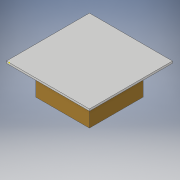
# Autodesk Inventor part: PartStoreipt
Saved by Autodesk Inventor 2018 (Build 220112000, 112)
## iProperties
Created: 2018-06-08
Part Number: PartStoreipt
Material: Generic
Document SubType Name: Modeling
Designer: 3400746
Density: 1 g/cm^3
Appearance: Default
Author: 3400746
Autodesk Inventor part; units mm, degrees
ref_plane "YZ Plane" through (0, 0, 0) normal (1, 0, 0) x (0, 1, 0)
ref_plane "XZ Plane" through (0, 0, 0) normal (0, 1, 0) x (-1, 0, 0)
ref_plane "XY Plane" through (0, 0, 0) normal (0, 0, 1) x (1, 0, 0)
sketch "Sketch1" plane through (0, 0, 0) normal (0, 1, 0) x (-1, 0, 0)
  line L0 (0, 0) -> (2159, 0)
  line L1 (2159, 0) -> (2159, -2159)
  line L2 (2159, -2159) -> (0, -2159)
  line L3 (0, -2159) -> (0, 0)
  dimension "d0" = 2159
  dimension "d1" = 2159
  dimension "d2" = 2159
  constraints: 8 end point, 2 perpendicular, 1 horizontal
  measures "d0" distance of L0.start L0.end
  measures "d1" distance of L0.end L1.end
  measures "d2" distance of L1.end L2.end
extrude "Extrusion1" add sketch "Sketch1" against normal blind 50.8
sketch "Sketch2" plane through (0, -50.8, 0) normal (0, -1, 0) x (1, 0, 0)
  line L0 (0, 0) -> (-2159, 0) projected
  line L1 (0, 0) -> (0, -381)
  line L2 (0, -2159) -> (0, 0) projected
  line L3 (-381, -381) -> (-381, -1778)
  line L4 (-381, -1778) -> (-1778, -1778)
  line L5 (-1778, -1778) -> (-1778, -381)
  line L6 (-1778, -381) -> (-381, -381)
  dimension "d7" = 1397
  dimension "d8" = 1397
  dimension "d9" = 1397
  constraints: 10 end point, 1 perpendicular, 1 point on line
  measures "d7" distance of L3.start L3.end
  measures "d8" distance of L3.end L4.end
  measures "d9" distance of L4.end L5.end
extrude "Extrusion2" add sketch "Sketch2" along normal blind 762
sketch "Sketch3" plane through (0, -50.8, 0) normal (0, -1, 0) x (1, 0, 0)
  line L0 (-2159, -2159) -> (0, -2159) projected
  line L1 (-2159, -2159) -> (-1934.4936, -1934.4936)
  line L2 (-2159, -2159) -> (-1841.5, -2159) construction
  circle A0 centre (-1934.4936, -1934.4936) radius 101.6
  point P0 (0, 0)
  dimension "d12" = 317.5
  dimension "d13" = 45
  dimension "d14" = 203.2
  constraints: 4 end point, 1 centre point, 1 coincident, 1 equal length, 1 horizontal
  measures "d12" distance of L0.start L1.end
  measures "d13" angle of L2 L1
  measures "d14" diameter of A0
extrude "Extrusion3" add sketch "Sketch3" along normal blind 1016
sketch "Sketch4" plane through (-1934.4936, -1066.8, -1934.4936) normal (0, -1, 0) x (1, 0, 0)
  line L0 (0, 0) -> (152.4, 0)
  line L1 (0, 0) -> (-152.4, 0)
  line L2 (152.4, 0) -> (152.4, -254)
  line L3 (152.4, 0) -> (152.4, 253.967)
  line L4 (156.4936, 156.4936) -> (156.4936, 1553.4936) projected
  line L5 (152.4, -254) -> (-152.4, -254)
  line L6 (-152.4, -254) -> (-152.4, 254)
  line L7 (152.4, 253.967) -> (-152.4, 254)
  point P0 (1934.4936, 1934.4936)
  dimension "d17" = 152.4
  dimension "d18" = 152.4
  dimension "d19" = 254
  dimension "d20" = 253.967
  dimension "d21" = 304.8
  dimension "d22" = 508
  constraints: 14 end point, 3 horizontal, 3 vertical, 1 other
  measures "d17" distance of L0.start L0.end
  measures "d18" distance of L0.start L1.end
  measures "d19" distance of L0.end L2.end
  measures "d20" distance of L0.end L3.end
  measures "d21" distance of L2.end L5.end
  measures "d22" distance of L5.end L6.end
extrude "Extrusion4" add sketch "Sketch4" along normal blind 254
sketch "Sketch5" plane through (-2086.8936, -1066.8, -2188.4936) normal (-1, 0, 0) x (0, 0, 1)
  point P0 (2188.4936, 1066.8)
sketch "Sketch6" plane through (-1778, -50.8, -1778) normal (-1, 0, 0) x (0, 0, 1)
  line L0 (0, 0) -> (127, 0)
  line L1 (0, 0) -> (1397, 0) projected
  line L2 (127, 0) -> (127, -762)
  line L3 (1397, 0) -> (1270, 0)
  line L4 (1270, 0) -> (1270, -762)
  line L5 (1270, -762) -> (1270, -635)
  line L6 (1270, -635) -> (127, -635)
  point P0 (1778, 50.8)
  dimension "d25" = 127
  dimension "d26" = 127
  dimension "d27" = 127
  constraints: 12 end point, 4 point on line, 2 vertical, 1 perpendicular
  measures "d25" distance of L0.start L0.end
  measures "d26" distance of L1.end L3.end
  measures "d27" distance of L4.end L5.end
extrude "Extrusion5" cut sketch "Sketch6" against normal blind 1270
sketch "Sketch7" plane through (-1778, -812.8, -1778) normal (-1, 0, 0) x (0, 0, 1)
  line L0 (0, 0) -> (0, 762)
  line L1 (-381, 762) -> (1778, 762) projected
  line L2 (0, 762) -> (698.5, 762)
  line L3 (698.5, 762) -> (698.5, 135.629)
  line L4 (698.5, 762) -> (825.5, 762)
  line L5 (1778, 762) -> (-381, 762) projected
  line L6 (698.5, 762) -> (571.5, 762)
  line L7 (825.5, 762) -> (825.5, 508)
  line L8 (825.5, 508) -> (571.5, 508)
  line L9 (571.5, 762) -> (571.5, 508)
  point P0 (1778, 812.8)
  dimension "d30" = 698.5
  dimension "d31" = 127
  dimension "d32" = 127
  dimension "d38" = 254
  dimension "d39" = 254
  constraints: 16 end point, 3 point on line, 3 vertical, 1 horizontal, 1 midpoint
  measures "d30" distance of L0.end L2.end
  measures "d31" distance of L2.end L4.end
  measures "d32" distance of L2.end L6.end
  measures "d38" distance of L4.end L7.end
  measures "d39" distance of L7.end L8.end
extrude "Extrusion6" add sketch "Sketch7" against normal blind 127
sketch "Sketch8" plane through (-1778, -812.8, -1778) normal (-1, 0, 0) x (0, 0, 1)
  line L0 (800.1, 533.4) -> (596.9, 533.4)
  line L1 (596.9, 533.4) -> (596.9, 762)
  line L2 (571.5, 762) -> (825.5, 762) projected
  line L3 (800.1, 533.4) -> (800.1, 762)
  point P0 (1778, 812.8)
  point P1 (825.5, 508)
  constraints: 6 end point, 2 point on line, 1 horizontal, 1 perpendicular, 1 vertical
extrude "Extrusion7" cut sketch "Sketch8" against normal blind 127
sketch "Sketch9" plane through (-1778, -812.8, -1778) normal (-1, 0, 0) x (0, 0, 1)
  line L0 (1047.75, 762) -> (1047.75, 127)
  line L1 (1270, 127) -> (127, 127) projected
  line L2 (1047.75, 762) -> (1111.25, 762)
  line L3 (1047.75, 762) -> (984.25, 762)
  line L4 (1111.25, 762) -> (1111.25, 127)
  line L5 (984.25, 762) -> (984.25, 127)
  line L6 (347.3726, 762) -> (283.8726, 762)
  line L7 (347.3726, 762) -> (410.8726, 762)
  line L8 (410.8726, 762) -> (410.8726, 127)
  line L9 (283.8726, 762) -> (283.8726, 127)
  line L10 (1270, 762) -> (1270, 127) projected
  line L11 (1270, 444.5) -> (1270, 508)
  line L12 (1270, 444.5) -> (1270, 381)
  line L13 (1270, 381) -> (127, 381)
  line L14 (127, 127) -> (127, 762) projected
  line L15 (1270, 508) -> (127, 508)
  point P0 (1778, 812.8)
  point P1 (825.5, 762)
  dimension "d48" = 63.5
  dimension "d49" = 63.5
  dimension "d51" = 63.5
  dimension "d52" = 63.5
  dimension "d53" = 635
  dimension "d55" = 63.5
  dimension "d56" = 63.5
  constraints: 26 end point, 9 point on line, 5 horizontal, 2 perpendicular, 2 vertical, 1 midpoint
  measures "d48" distance of L0.start L2.end
  measures "d49" distance of L0.start L3.end
  measures "d51" distance of L6.start L6.end
  measures "d52" distance of L6.start L7.end
  measures "d53" distance of L6.end L9.end
  measures "d55" distance of L11.start L11.end
  measures "d56" distance of L11.start L12.end
extrude "Extrusion8" add sketch "Sketch9" against normal blind 127 contours L2 L4 L15 L0 | L0 L15 L5 L3 | L15 L4 L13 L0 | L0 L13 L5 L15 | L13 L4 L1 L0 | L0 L1 L5 L13 | L15 L10 L13 L4 | L5 L13 L8 L15 | L15 L9 L6 L7 L8 | L8 L13 L9 L15 | L8 L1 L9 L13 | L9 L13 L14 L15
sketch "Sketch10" plane through (0, -50.8, 0) normal (0, -1, 0) x (1, 0, 0)
  line L0 (-1778, -508) -> (-1778, -381) projected
  line L1 (-1778, -381) -> (-1778, -1778)
  line L2 (-381, -381) -> (-381, -1778) projected
  line L3 (-1778, -1778) -> (-381, -1778)
  line L4 (-381, -381) -> (-1778, -381) projected
  line L5 (-381, -1778) -> (-381, -381)
  line L6 (-381, -381) -> (-1778, -381)
  point P0 (0, 0)
  dimension "d59" = 1397
  dimension "d60" = 1397
  constraints: 8 end point, 2 collinear, 1 vertical
  measures "d59" distance of L0.end L1.end
  measures "d60" distance of L2.start L0.end
extrude "Extrusion9" add sketch "Sketch10" along normal blind 2.54
body "Solid1"
